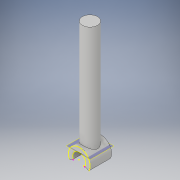
# Autodesk Inventor part: golf1
Saved by Autodesk Inventor 2018.3 (Build 223284000, 284)
## iProperties
Created: 2019-05-03
Part Number: golf1
Material: Generic
Document SubType Name: Modeling
Designer: F8PLTW
Density: 1 g/cm^3
Appearance: Default
Author: F8PLTW
Autodesk Inventor part; units mm, degrees
ref_plane "YZ Plane" through (0, 0, 0) normal (1, 0, 0) x (0, 1, 0)
ref_plane "XZ Plane" through (0, 0, 0) normal (0, 1, 0) x (-1, 0, 0)
ref_plane "XY Plane" through (0, 0, 0) normal (0, 0, 1) x (1, 0, 0)
sketch "Sketch1" plane through (0, 0, 0) normal (0, 0, 1) x (1, 0, 0)
  arc A0 (6.1036, -1.9996) -> (-16.8874, -1.4338) centre (-5.2593, 3.6728) ccw
  arc A1 (1.5584, 0.2694) -> (-12.2361, 0.6088) centre (-5.2593, 3.6728) ccw
  line L0 (-12.2361, 0.6088) -> (-16.8874, -1.4338)
  line L1 (1.5584, 0.2694) -> (6.1036, -1.9996)
  point P0 (0, 0)
  dimension "d0" = 25.4
  dimension "d1" = 15.24
  constraints: 4 end point, 4 point on circle, 2 centre point, 1 coincident
  measures "d0" diameter of A0
  measures "d1" diameter of A1
extrude "Extrusion1" add sketch "Sketch1" along normal blind 25.4
sketch "Sketch2" plane through (0, 0, 25.4) normal (0, 0, 1) x (1, 0, 0)
  arc A0 (6.1036, -1.9996) -> (-16.8874, -1.4338) centre (-5.2593, 3.6728) ccw projected
  line L0 (-5.2593, 16.3728) -> (1.9559, 16.3728) construction
  arc A1 (1.5584, 0.2694) -> (-12.2361, 0.6088) centre (-5.2593, 3.6728) ccw projected
  line L1 (-5.2593, 11.2928) -> (0.7923, 11.2928) construction
  point P0 (0, 0)
  point P1 (-12.1004, 0.3168)
  point P2 (1.2826, -0.2347)
  constraints: 4 end point, 2 horizontal, 2 point on circle, 2 tangent
ref_plane "Work Plane2" through (-5.2593, 11.2928, 25.4) normal (0, -1, 0) x (1, 0, 0)
sketch "Sketch3" plane through (-5.2593, 11.2928, 25.4) normal (0, -1, 0) x (1, 0, 0)
  line L0 (12.7, 0) -> (-12.7, 0) projected
  line L1 (-12.7, -25.4) -> (12.7, -25.4) projected
  line L2 (-12.7, 0) -> (12.7, -25.4) construction
  line L3 (12.7, 0) -> (-12.7, -25.4) construction
  circle A0 centre (0, -12.7) radius 8.89
  point P0 (5.2593, -25.4)
  point P1 (11.3628, 0)
  point P2 (-11.6281, 0)
  point P3 (11.3628, -25.4)
  point P4 (-11.6281, -25.4)
  dimension "d4" = 17.78
  constraints: 4 end point, 1 centre point, 1 midpoint
  measures "d4" diameter of A0
extrude "Extrusion2" add sketch "Sketch3" against normal blind 127
body "Solid1"
